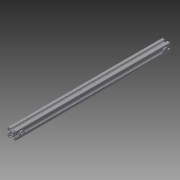
# Autodesk Inventor part: Lift Section
Saved by Autodesk Inventor 2013 (Build 170138000, 138)
## iProperties
Created: 2014-09-14
Part Number: Lift Section
Document SubType Name: Modeling
Designer: Family Room
Density: 1 g/cm^3
Material: Generic
Author: Family Room
Autodesk Inventor part; units mm, degrees
sketch "Sketch1" plane through (0, 0, 0) normal (0, 0, 1) x (1, 0, 0)
  line L0 (0.1212, -19.5) -> (-0.3333, -19.5)
  line L1 (0.1212, -20) -> (0.1212, -19.5)
  line L2 (5.1624, -20) -> (0.1212, -20)
  arc A0 (5.1624, -20) -> (6.6667, -18.4957) centre (5.1624, -18.4957) ccw
  line L3 (6.6667, -13.3333) -> (6.6667, -18.4957)
  line L4 (6.2121, -13.3333) -> (6.6667, -13.3333)
  line L5 (6.2121, -13) -> (6.2121, -13.3333)
  line L6 (5.0758, -13) -> (6.2121, -13)
  line L7 (5.0758, -16) -> (5.0758, -13)
  line L8 (3.7121, -16) -> (5.0758, -16)
  line L9 (1.2121, -13.3333) -> (3.7121, -16)
  line L10 (1.2121, -10.8302) -> (1.2121, -13.3333)
  arc A1 (1.2121, -9.1698) -> (1.2121, -10.8302) centre (1.483, -10) ccw
  line L11 (1.2121, -6.5455) -> (1.2121, -9.1698)
  line L12 (3.6667, -4.0909) -> (1.2121, -6.5455)
  line L13 (5.1667, -4.0909) -> (3.6667, -4.0909)
  line L14 (5.1667, -7) -> (5.1667, -4.0909)
  line L15 (6.1667, -7) -> (5.1667, -7)
  line L16 (6.1667, -6.5455) -> (6.1667, -7)
  line L17 (6.6667, -6.5455) -> (6.1667, -6.5455)
  line L18 (6.6667, -1.5043) -> (6.6667, -6.5455)
  arc A2 (6.6667, -1.5043) -> (5.1624, 0) centre (5.1624, -1.5043) ccw
  line L19 (0, 0) -> (5.1624, 0)
  line L20 (0, -0.4545) -> (0, 0)
  line L21 (-0.3333, -0.4545) -> (0, -0.4545)
  line L22 (-0.3333, -1.5909) -> (-0.3333, -0.4545)
  line L23 (2.6667, -1.5909) -> (-0.3333, -1.5909)
  line L24 (2.6667, -2.9545) -> (2.6667, -1.5909)
  line L25 (0, -5.4545) -> (2.6667, -2.9545)
  line L26 (-2.5032, -5.4545) -> (0, -5.4545)
  arc A3 (-4.1635, -5.4545) -> (-2.5032, -5.4545) centre (-3.3333, -5.1837) ccw
  line L27 (-6.7879, -5.4545) -> (-4.1635, -5.4545)
  line L28 (-9.2424, -3) -> (-6.7879, -5.4545)
  line L29 (-9.2424, -1.5) -> (-9.2424, -3)
  line L30 (-6.3333, -1.5) -> (-9.2424, -1.5)
  line L31 (-6.3333, -0.5) -> (-6.3333, -1.5)
  line L32 (-6.7879, -0.5) -> (-6.3333, -0.5)
  line L33 (-6.7879, 0) -> (-6.7879, -0.5)
  line L34 (-11.829, 0) -> (-6.7879, 0)
  arc A4 (-11.829, 0) -> (-13.3333, -1.5043) centre (-11.829, -1.5043) ccw
  line L35 (-13.3333, -6.6667) -> (-13.3333, -1.5043)
  line L36 (-12.8788, -6.6667) -> (-13.3333, -6.6667)
  line L37 (-12.8788, -7) -> (-12.8788, -6.6667)
  line L38 (-11.7424, -7) -> (-12.8788, -7)
  line L39 (-11.7424, -4) -> (-11.7424, -7)
  line L40 (-10.3788, -4) -> (-11.7424, -4)
  line L41 (-7.8788, -6.6667) -> (-10.3788, -4)
  line L42 (-7.8788, -9.1698) -> (-7.8788, -6.6667)
  arc A5 (-7.8788, -10.8302) -> (-7.8788, -9.1698) centre (-8.1497, -10) ccw
  line L43 (-7.8788, -13.4545) -> (-7.8788, -10.8302)
  line L44 (-10.3333, -15.9091) -> (-7.8788, -13.4545)
  line L45 (-11.8333, -15.9091) -> (-10.3333, -15.9091)
  line L46 (-11.8333, -13) -> (-11.8333, -15.9091)
  line L47 (-12.8333, -13) -> (-11.8333, -13)
  line L48 (-12.8333, -13.4545) -> (-12.8333, -13)
  line L49 (-13.3333, -13.4545) -> (-12.8333, -13.4545)
  line L50 (-13.3333, -18.4957) -> (-13.3333, -13.4545)
  arc A6 (-13.3333, -18.4957) -> (-11.829, -20) centre (-11.829, -18.4957) ccw
  line L51 (-6.6667, -20) -> (-11.829, -20)
  line L52 (-6.6667, -19.5455) -> (-6.6667, -20)
  line L53 (-6.3333, -19.5455) -> (-6.6667, -19.5455)
  line L54 (-6.3333, -18.4091) -> (-6.3333, -19.5455)
  line L55 (-9.3333, -18.4091) -> (-6.3333, -18.4091)
  line L56 (-9.3333, -17.0455) -> (-9.3333, -18.4091)
  line L57 (-6.6667, -14.5455) -> (-9.3333, -17.0455)
  line L58 (-4.1635, -14.5455) -> (-6.6667, -14.5455)
  arc A7 (-2.5032, -14.5455) -> (-4.1635, -14.5455) centre (-3.3333, -14.8163) ccw
  line L59 (0.1212, -14.5455) -> (-2.5032, -14.5455)
  line L60 (2.5758, -17) -> (0.1212, -14.5455)
  line L61 (2.5758, -18.5) -> (2.5758, -17)
  line L62 (-0.3333, -18.5) -> (2.5758, -18.5)
  line L63 (-0.3333, -19.5) -> (-0.3333, -18.5)
  line L64 (-1.523, -12.9923) -> (-2.0717, -12.4435)
  arc A8 (-4.5949, -12.4435) -> (-2.0717, -12.4435) centre (-3.3333, -10) ccw
  line L65 (-4.5949, -12.4435) -> (-5.1437, -12.9923)
  line L66 (-5.1437, -12.9923) -> (-6.3256, -11.8104)
  line L67 (-6.3256, -11.8104) -> (-5.7769, -11.2616)
  arc A9 (-5.7769, -8.7384) -> (-5.7769, -11.2616) centre (-3.3333, -10) ccw
  line L68 (-5.7769, -8.7384) -> (-6.3256, -8.1896)
  line L69 (-6.3256, -8.1896) -> (-5.1437, -7.0077)
  line L70 (-5.1437, -7.0077) -> (-4.5949, -7.5565)
  arc A10 (-2.0717, -7.5565) -> (-4.5949, -7.5565) centre (-3.3333, -10) ccw
  line L71 (-2.0717, -7.5565) -> (-1.523, -7.0077)
  line L72 (-1.523, -7.0077) -> (-0.3411, -8.1896)
  line L73 (-0.3411, -8.1896) -> (-0.8898, -8.7384)
  arc A11 (-0.8898, -11.2616) -> (-0.8898, -8.7384) centre (-3.3333, -10) ccw
  line L74 (-0.8898, -11.2616) -> (-0.3411, -11.8104)
  line L75 (-0.3411, -11.8104) -> (-1.523, -12.9923)
  point P0 (-13.3333, -20)
  constraints: 152 end point, 24 point on circle, 12 centre point
extrude "Extrusion1" add sketch "Sketch1" along normal mid plane 374.65
ref_plane "Work Plane1" through (-3.3333, -6.5455, 187.325) normal (1, 0, 0) x (0, 0, -1)
ref_plane "Work Plane2" through (-6.7879, -10, 187.325) normal (0, 1, 0) x (1, 0, 0)
sketch "Sketch2" plane through (-6.3333, -0.5, 187.325) normal (0, 1, 0) x (1, 0, 0)
  line L0 (0, 0) -> (0, 374.65) projected
  line L1 (0, 374.65) -> (-0.4545, 374.65) projected
  line L2 (-5.4957, 0) -> (-0.4545, 0) projected
  point P0 (6.3333, 187.325)
  point P1 (3, 171.45)
  point P2 (3, 203.2)
  dimension "d2" = 3
  dimension "d3" = 203.2
  dimension "d11" = 203.2
  measures "d2" distance from line of L0 point (3, 171.45)
  measures "d3" distance from line of L1 point (3, 171.45)
  measures "d11" distance from line of L2 point (3, 203.2)
hole "Hole1" at (-3.3333, -0.5, 15.875) at (-3.3333, -0.5, -15.875) direction (0, -1, 0) diameter 6.35 end through all
ref_plane "Work Plane3" through (6.6667, -13.3333, -187.325) normal (1, 0, 0) x (0, 0, -1)
sketch "Sketch3" plane through (6.6667, -13.3333, -187.325) normal (1, 0, 0) x (0, 0, -1)
  circle A0 centre (-12.7, 3.3333) radius 6.35
  circle A1 centre (-361.95, 3.3333) radius 6.35
  line L0 (-374.65, -6.6667) -> (0, -6.6667) projected
  line L1 (-374.65, 11.829) -> (-374.65, 6.7879) projected
  line L2 (0, 6.7879) -> (0, 11.829) projected
  point P0 (-187.325, 13.3333)
  dimension "d12" = 12.7
  dimension "d13" = 12.7
  dimension "d14" = 10
  dimension "d15" = 12.7
  dimension "d16" = 12.7
  dimension "d17" = 10
  constraints: 2 centre point
  measures "d12" diameter of A0
  measures "d13" diameter of A1
  measures "d14" distance from line of L0 A1.centre
  measures "d15" distance from line of L1 A1.centre
  measures "d16" distance from line of L2 A0.centre
  measures "d17" distance from line of L0 A0.centre
extrude "Extrusion2" add sketch "Sketch3" along normal blind 2.54
sketch "Sketch4" plane through (9.2067, -10, 174.625) normal (1, 0, 0) x (0, 0, -1)
  circle A0 centre (0, 0) radius 6.35 projected
  circle A1 centre (0, 0) radius 3.175
  circle A2 centre (355.6, 0) radius 3.175
  point P0 (174.625, 10)
  dimension "d20" = 6.35
  dimension "d21" = 355.6
  dimension "d22" = 0
  dimension "d23" = 6.35
  constraints: 3 coincident, 2 centre point
  measures "d20" diameter of A1
  measures "d21" distance of point (355.6, 0) A1.centre
  measures "d22" vertical distance of A0.centre point (355.6, 0)
  measures "d23" diameter of A2
extrude "Extrusion3" add sketch "Sketch4" along normal blind 2.54 contours A1 | A2
body "Solid1"
